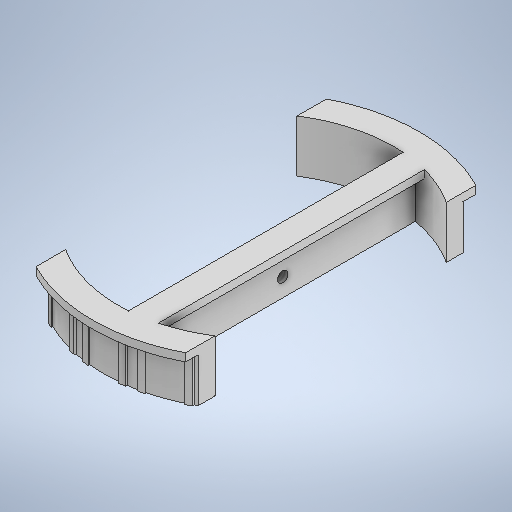
# Autodesk Inventor part: Part2
Saved by Autodesk Inventor 2025 (Build 290162010, 162A)
## iProperties
Created: 2024-06-17
Part Number: Part2
Material: Generic
Document SubType Name: Modeling
Designer: vncnt
Density: 1 g/cm^3
Appearance: Default
Author: vncnt
## iProperties of the stored document AQS_Mount_3DPrint.ipt
Created: 2024-06-27
Part Number: AQS_Mount_3DPrint
Material: Generic
Document SubType Name: Modeling
Designer: vncnt
Density: 1 g/cm^3
Appearance: Default
Author: vncnt
Autodesk Inventor part; units mm, degrees
ref_plane "YZ Plane" through (0, 0, 0) normal (1, 0, 0) x (0, 1, 0)
ref_plane "XZ Plane" through (0, 0, 0) normal (0, 1, 0) x (-1, 0, 0)
ref_plane "XY Plane" through (0, 0, 0) normal (0, 0, 1) x (1, 0, 0)
sketch "Sketch1" plane through (0, 0, 0) normal (0, 1, 0) x (-1, 0, 0)
  circle A0 centre (0, 0) radius 38.65
  circle A1 centre (0, 0) radius 23.65
  line L0 (19, 63) -> (-19, 63)
  line L1 (-19, 63) -> (-19, -63)
  line L2 (-19, -63) -> (19, -63)
  line L3 (19, -63) -> (19, 63)
  line L4 (19, 63) -> (-19, -63) construction
  line L5 (-19, 63) -> (19, -63) construction
  point P0 (19, -33.6574)
  point P1 (19, -14.0827)
  point P2 (-19, -14.0827)
  point P3 (-19, -33.6574)
  point P4 (19, 14.0827)
  point P5 (19, 33.6574)
  point P6 (-19, 33.6574)
  point P7 (-19, 14.0827)
  dimension "d0" = 77.3
  dimension "d1" = 15
  constraints: 12 end point, 2 centre point, 2 midpoint, 2 parallel, 1 coincident, 1 horizontal, 1 perpendicular
  measures "d0" diameter of A0
  measures "d1" radial gap between concentric circles of A0 A1
extrude "Extrusion1" add sketch "Sketch1" along normal blind 25 contours L3 A1 L1 A0 | A0 L1 A1 L3
sketch "Sketch2" plane through (0, 25, 0) normal (0, 1, 0) x (1, 0, 0)
  line L0 (-2.5, -27.5) -> (2.5, -27.5)
  line L1 (2.5, -27.5) -> (2.5, 27.5)
  line L2 (2.5, 27.5) -> (-2.5, 27.5)
  line L3 (-2.5, 27.5) -> (-2.5, -27.5)
  line L4 (-2.5, -27.5) -> (2.5, 27.5) construction
  line L5 (2.5, -27.5) -> (-2.5, 27.5) construction
  line L6 (-7, -32) -> (7, -32)
  line L7 (7, -32) -> (7, 32)
  line L8 (7, 32) -> (-7, 32)
  line L9 (-7, 32) -> (-7, -32)
  line L10 (-9.7051, -15.4838) -> (-1.8651, -15.4838)
  line L11 (-1.8651, -15.4838) -> (-1.8651, 20.5162)
  line L12 (-1.8651, 20.5162) -> (-9.7051, 20.5162)
  line L13 (-9.7051, 20.5162) -> (-9.7051, -15.4838)
  line L14 (-9.7051, -15.4838) -> (-1.8651, 20.5162) construction
  line L15 (-1.8651, -15.4838) -> (-9.7051, 20.5162) construction
  point P0 (0, 0)
  point P1 (-5.7851, 2.5162)
  dimension "d4" = 5
  dimension "d5" = 55
  constraints: 32 end point, 6 parallel, 4 midpoint, 3 perpendicular, 2 horizontal, 1 point on line, 3 other
  measures "d4" distance of L1.end L2.end
  measures "d5" distance of L0.end L1.end
extrude "Extrusion2" cut sketch "Sketch2" against normal through all contours L3 L10 L11 L12 L2 L1 L0 | L3 L12 L11 L10
sketch "Sketch3" plane through (0, 25, 0) normal (0, 1, 0) x (1, 0, 0)
  line L0 (2.5, 27.5) -> (2.5, 23.5175) projected
  line L1 (-2.5, -27.5) -> (2.5, -27.5)
  line L2 (2.5, -27.5) -> (2.5, 27.5)
  line L3 (2.5, 27.5) -> (-2.5, 27.5)
  line L4 (-2.5, 27.5) -> (-2.5, -27.5)
  line L5 (-2.5, -27.5) -> (2.5, 27.5) construction
  line L6 (2.5, -27.5) -> (-2.5, 27.5) construction
  line L7 (6, 31) -> (6, -31)
  line L8 (6, -31) -> (-6, -31)
  line L9 (-6, -31) -> (-6, 31)
  line L10 (-6, 31) -> (6, 31)
  line L11 (-9.5, -20) -> (-2.5, -20)
  line L12 (-2.5, -20) -> (-2.5, 20)
  line L13 (-2.5, 20) -> (-9.5, 20)
  line L14 (-9.5, 20) -> (-9.5, -20)
  line L15 (-9.5, -20) -> (-2.5, 20) construction
  line L16 (-2.5, -20) -> (-9.5, 20) construction
  point P0 (0, 0)
  point P1 (-6, 0)
  point P2 (-2.5, -20)
  point P3 (-6, -20)
  point P4 (-6, 20)
  constraints: 32 end point, 6 parallel, 4 midpoint, 3 perpendicular, 2 horizontal, 1 point on line, 3 other
extrude "Extrusion3" add sketch "Sketch3" against normal up to surface (25 mm away) contours L3 L4 L13 L9 L10 L7 L8 L11 L1 L2 L0
sketch "Sketch9" plane through (0, 0, 0) normal (0, 1, 0) x (-1, 0, 0)
  circle A0 centre (0, 0) radius 39.05
  circle A1 centre (0, 0) radius 37.4109
  line L0 (18.3198, 40.4963) -> (-18.3198, 40.4963)
  line L1 (-18.3198, 40.4963) -> (-18.3198, -40.4963)
  line L2 (-18.3198, -40.4963) -> (18.3198, -40.4963)
  line L3 (18.3198, -40.4963) -> (18.3198, 40.4963)
  line L4 (18.3198, 40.4963) -> (-18.3198, -40.4963) construction
  line L5 (-18.3198, 40.4963) -> (18.3198, -40.4963) construction
  line L6 (-18.3198, -38.5344) -> (-16.924, -38.5344)
  line L7 (-16.924, -38.5344) -> (-16.924, 37.4109)
  line L8 (-16.924, 37.4109) -> (-18.3198, 37.4109)
  line L9 (-18.3198, 37.4109) -> (-18.3198, -38.5344)
  point P0 (18.3198, -34.4861)
  point P1 (18.3198, -32.6184)
  point P2 (-18.3198, -32.6184)
  point P3 (-18.3198, -34.4861)
  point P4 (18.3198, 32.6184)
  point P5 (18.3198, 34.4861)
  point P6 (-18.3198, 34.4861)
  point P7 (-18.3198, 32.6184)
  point P8 (-16.924, -35.1921)
  point P9 (-16.924, -33.3639)
  point P10 (-16.924, 33.3639)
  point P11 (-16.924, 35.1921)
  dimension "d31" = 78.1
  constraints: 20 end point, 4 parallel, 2 centre point, 2 coincident, 2 horizontal, 2 midpoint, 2 perpendicular, 2 point on line
  measures "d31" diameter of A0
extrude "Extrusion5" add sketch "Sketch9" along normal up to surface (25 mm away) contours L7 A1 L1 A0 | A0 L1 A1 L7
pattern_circular "Circular Pattern1" count 18 over 360 about axis through (0, -10, 0) along (0, 1, 0) of "Extrusion5"
sketch "Sketch11" plane through (0, 25, 0) normal (0, 1, 0) x (1, 0, 0)
  line L0 (-19, 33.6574) -> (-19, 14.0827) projected
  line L1 (-19, 33.6574) -> (-53, 33.6574)
  line L2 (-53, 33.6574) -> (-53, -45.1721)
  line L3 (-53, -45.1721) -> (-19, -45.1721)
  line L4 (-19, -45.1721) -> (-19, 33.6574)
  line L5 (19, 33.6574) -> (57, 33.6574)
  line L6 (57, 33.6574) -> (57, -45.1721)
  line L7 (57, -45.1721) -> (19, -45.1721)
  line L8 (19, -45.1721) -> (19, 33.6574)
  point P0 (0, 0)
  constraints: 16 end point, 4 parallel, 2 horizontal, 2 perpendicular, 2 point on line
extrude "Extrusion6" cut sketch "Sketch11" against normal through all
sketch "Sketch12" plane through (0, 25, 0) normal (0, 1, 0) x (1, 0, 0)
  circle A0 centre (0, 0) radius 41.5
  line L0 (-19, -51) -> (19, -51)
  line L1 (19, -51) -> (19, 51)
  line L2 (19, 51) -> (-19, 51)
  line L3 (-19, 51) -> (-19, -51)
  line L4 (-19, -51) -> (19, 51) construction
  line L5 (19, -51) -> (-19, 51) construction
  circle A1 centre (0, 0) radius 23.65
  line L6 (2.5, 30) -> (-2.5, 30)
  line L7 (-2.5, 30) -> (-2.5, -30)
  line L8 (-2.5, -30) -> (2.5, -30)
  line L9 (2.5, -30) -> (2.5, 30)
  line L10 (2.5, 30) -> (-2.5, -30) construction
  line L11 (-2.5, 30) -> (2.5, -30) construction
  line L12 (6, 22.8762) -> (6, -22.8762) projected
  line L13 (6, 22.8762) -> (6, -22.8762)
  line L14 (6, 22.8762) -> (9, 22.8762)
  line L15 (9, 22.8762) -> (9, -24.1579)
  line L16 (9, -24.1579) -> (6, -24.1579)
  line L17 (6, -24.1579) -> (6, 22.8762)
  line L18 (9, 22.8762) -> (6, 22.8762)
  line L19 (6, 22.8762) -> (6, 28)
  line L20 (6, 28) -> (9, 28)
  line L21 (9, 28) -> (9, 22.8762)
  point P0 (-19, 36.8951)
  point P1 (-19, -36.8951)
  point P2 (19, -36.8951)
  point P3 (19, 36.8951)
  point P4 (2.5, -27.5)
  point P5 (19, 14.0827)
  point P6 (19, -14.0827)
  point P7 (-2.5, -23.5175)
  point P8 (-2.5, 23.5175)
  point P9 (2.5, 23.5175)
  point P10 (2.5, -23.5175)
  point P11 (9, -21.8706)
  point P12 (9, 21.8706)
  point P13 (-19, 14.0827)
  point P14 (-19, -14.0827)
  dimension "d42" = 83
  dimension "d52" = 60
  constraints: 42 end point, 9 equal length, 4 horizontal, 4 midpoint, 4 perpendicular, 2 centre point, 2 point on line, 1 coincident, 1 point on circle
  measures "d42" diameter of A0
  measures "d52" distance of L7.end L6.end
extrude "Extrusion7" add sketch "Sketch12" along normal blind 2 contours L1 A1 L15 L21 L20 L19 L9 L6 L7 L3 A0 | A0 L3 A1 L7 L8 L9 L17 L16 L15 L1 | L15 A1 L12 | A1 L14 L15 | L15 L16 L17 A1 | L7 L6 L9 A1 | A1 L9 L7 | L12 A1 L9 | L19 L20 L21 L14 | A1 L9 L8 L7
sketch "Sketch14" plane through (0, 0, 0) normal (0, -1, 0) x (1, 0, 0)
  circle A0 centre (0, 0) radius 54.8179
  constraints: 1 centre point, 1 coincident
extrude "Extrusion9" cut sketch "Sketch14" against normal blind 13.75
sketch "Sketch18" plane through (0, 25, 0) normal (0, -1, 0) x (1, 0, 0)
  circle A0 centre (0, 0) radius 35
  line L0 (-2.5, -23.5175) -> (-2.5, -27.5) projected
  line L1 (6, -27.5) -> (6, -45)
  line L2 (6, -45) -> (-2.5, -45)
  line L3 (-2.5, -45) -> (-2.5, -27.5)
  line L4 (6, -27.5) -> (6, 15)
  line L5 (-2.5, 15) -> (-2.5, -27.5)
  line L6 (6, 15) -> (6, 45)
  line L7 (6, 45) -> (-2.5, 45)
  line L8 (-2.5, 45) -> (-2.5, 15)
  line L9 (6, 45) -> (6, -45)
  line L10 (9, 21.8706) -> (9, -21.8706) projected
  line L11 (9, 0) -> (9, -45.2857)
  line L12 (9, -45.2857) -> (9, 53)
  point P0 (-2.5, 34.9106)
  point P1 (-2.5, -34.9106)
  point P2 (6, 34.4819)
  point P3 (6, -34.4819)
  point P4 (9, 33.8231)
  point P5 (9, -33.8231)
  dimension "d62" = 70
  constraints: 22 end point, 3 parallel, 3 point on line, 2 collinear, 1 centre point, 1 coincident, 1 midpoint
  measures "d62" diameter of A0
extrude "Extrusion13" cut sketch "Sketch18" along normal through all both and the other way through all contours A0 L11 L10 L12 | L8 L5 L0 L3 A0
sketch "Sketch19" plane through (0, 13.75, 0) normal (0, -1, 0) x (1, 0, 0)
  line L0 (-2.5, -27.5) -> (2.5, -27.5) projected
  line L1 (-2.5, -27.5) -> (2.5, -27.5)
  line L2 (2.5, -27.5) -> (2.5, -34.9106)
  line L3 (-2.5, -34.9106) -> (-2.5, -27.5)
  line L4 (-2.5, 27.5) -> (2.5, 27.5)
  line L5 (2.5, 27.5) -> (2.5, 34.9106)
  line L6 (-2.5, 34.9106) -> (-2.5, 27.5)
  arc A0 (-2.5, -34.9106) -> (2.5, -34.9106) centre (0, 0) ccw
  arc A1 (2.5, 34.9106) -> (-2.5, 34.9106) centre (0, 0) ccw
  line L7 (19, 36.8951) -> (19, 29.3939) projected
  line L8 (-19, 29.3939) -> (-19, 33.6574) projected
  arc A2 (19, 29.3939) -> (-19, 29.3939) centre (0, 0) ccw
  line L9 (19, -29.3939) -> (19, -33.6574) projected
  arc A3 (-19, -29.3939) -> (19, -29.3939) centre (0, 0) ccw
  arc A4 (9, 21.8706) -> (6, 22.8762) centre (0, 0) ccw projected
  line L10 (6, 22.8762) -> (11, 22.8762)
  line L11 (11, 22.8762) -> (11, 36)
  line L12 (11, 36) -> (6, 36)
  line L13 (6, 36) -> (6, 22.8762)
  line L14 (11, 22.8762) -> (6, 22.8762)
  line L15 (6, 22.8762) -> (6, 18)
  line L16 (6, 18) -> (11, 18)
  line L17 (11, 18) -> (11, 22.8762)
  arc A5 (6, -22.8762) -> (9, -21.8706) centre (0, 0) ccw projected
  line L18 (9, -21.8706) -> (6, -21.8706)
  line L19 (6, -21.8706) -> (6, -22.8762)
  line L20 (6, -22.8762) -> (9, -22.8762)
  line L21 (9, -22.8762) -> (9, -21.8706)
  line L22 (6, -22.8762) -> (9, -22.8762)
  line L23 (9, -22.8762) -> (9, -42)
  line L24 (9, -42) -> (6, -42)
  line L25 (6, -42) -> (6, -22.8762)
  point P0 (2.5, -27.5)
  point P1 (11, 33.2265)
  point P2 (6, 34.4819)
  point P3 (6, -34.4819)
  point P4 (9, -33.8231)
  constraints: 44 end point, 10 parallel, 9 point on circle, 6 horizontal, 6 perpendicular, 4 centre point, 3 point on line, 2 concentric, 1 coincident
extrude "Extrusion14" cut sketch "Sketch19" against normal up to surface (11.25 mm away) contours L0 L2 A0 L3 | L6 A1 L5 L4 | L11 L10 L13 A2 | L17 L16 L15 L10 | L25 L20 L23 A3 | L19 L18 A5 | A5 L21 L20
sketch "Sketch20" plane through (2.5, 13.75, 34.9106) normal (-1, 0, 0) x (0, 0, 1)
  line L0 (0, 0) -> (0, 11.25) projected
  line L1 (-69.8212, 11.25) -> (0, 11.25) projected
  point P0 (-34.9106, -13.75)
  point P1 (-35.696, 4.646)
  dimension "d67" = 35.696
  dimension "d68" = 6.604
  measures "d67" distance from line of L0 point (-35.696, 4.646)
  measures "d68" distance from line of L1 point (-35.696, 4.646)
hole "Hole3" at (2.5, 18.396, -0.7854) direction (1, 0, 0) diameter 2.6416 depth 10.979 thread size "6-32 UNC" class "2B" standard "ANSI Unified Screw Threads"
sketch "Sketch21" plane through (0, 27, 0) normal (0, 1, 0) x (1, 0, 0)
  line L0 (2.5, -34.9106) -> (2.5, 34.9106)
  line L1 (-2.5, 34.9106) -> (-2.5, -34.9106)
  line L2 (2.5, -34.9106) -> (2.5, 34.9106)
  arc A0 (19, 29.3939) -> (9, 33.8231) centre (0, 0) ccw
  line L3 (-19, 36.8951) -> (-19, 29.3939) projected
  arc A1 (19, 29.3939) -> (-19, 29.3939) centre (0, 0) ccw
  arc A2 (-19, -29.3939) -> (19, -29.3939) centre (0, 0) ccw
  constraints: 9 point on circle, 6 end point, 3 centre point, 1 parallel
extrude "Extrusion15" cut sketch "Sketch21" against normal through all
body "Solid1"
